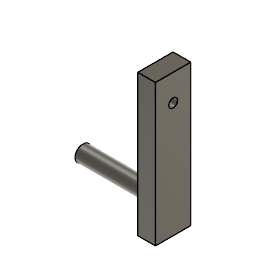
wheel base (Autodesk Fusion 360 design; units mm, degrees)
Autodesk Fusion 360 part; units mm, degrees
sketch "Sketch1" plane through (0, 0, 0) normal (0, 0, 1) x (1, 0, 0)
  line L0 (0, 0) -> (-10, 0)
  line L1 (-10, 0) -> (-10, 20)
  line L2 (-10, 20) -> (0, 20)
  line L3 (0, 20) -> (0, 0)
  constraint horizontal L0
  constraint vertical L1
  constraint horizontal L2
  constraint vertical L3
  constraint coincident L0.start L3.end
extrude "Extrude1" add sketch "Sketch1" along normal blind 80
sketch "Sketch2" plane through (-10, 0, 0) normal (-1, 0, 0) x (0, -1, 0)
  line L0 (-20, 0) -> (0, 0)
  line L1 (0, 80) -> (-20, 80)
  line L2 (-20, 80) -> (-20, 0)
  circle A0 centre (-10, 15) radius 4.5
  line L3 (-10, 15) -> (-10, 65)
  line L4 (0, 0) -> (0, 80)
  point P0 (-10, 65)
  dimension "d3" = 9
  dimension "d6" = 15
  dimension "d7" = 50
  dimension "d11" = 10
  constraint coincident A0.centre L3.start
  constraint perpendicular L1 L3
  constraint coincident P0 L3.end
  measures "d3" diameter of A0
  measures "d6" distance of L0 A0.centre
  measures "d7" distance of A0.centre P0
  measures "d11" distance of L2 A0.centre
extrude "Extrude2" add sketch "Sketch2" along normal blind 41 contours A0
hole "Hole1" at (-10, 10, 65) direction (1, 0, 0) diameter 5 depth 10 tip angle 118
